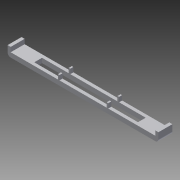
# Autodesk Inventor part: base_corner
Saved by Autodesk Inventor 2014 SP1 (Build 180222100, 222)
## iProperties
Created: 2016-08-31
Part Number: base_corner
Material: ABS Plastic
Document SubType Name: Modeling
Designer: tguillod
Density: 1.06 g/cm^3
Appearance: Smooth - White
Author: tguillod
Autodesk Inventor part; units mm, degrees
ref_plane "YZ Plane" through (0, 0, 0) normal (1, 0, 0) x (0, 1, 0)
ref_plane "XZ Plane" through (0, 0, 0) normal (0, 1, 0) x (-1, 0, 0)
ref_plane "XY Plane" through (0, 0, 0) normal (0, 0, 1) x (1, 0, 0)
sketch "Sketch1" plane through (0, 0, 0) normal (0, 0, 1) x (1, 0, 0)
  line L0 (0, 0) -> (97.5, 0)
  line L1 (97.5, 0) -> (97.5, 9)
  line L2 (97.5, 9) -> (0, 9)
  line L3 (0, 9) -> (0, 0)
  dimension "d2" = 97.5
  dimension "d3" = 9
  constraints: 8 end point, 2 parallel, 1 horizontal, 1 perpendicular
  measures "d2" distance of L1.end L2.end
  measures "d3" distance of L0.end L1.end
extrude "Extrusion1" add sketch "Sketch1" along normal blind 6
sketch "Sketch2" plane through (0, 0, 6) normal (0, 0, 1) x (1, 0, 0)
  line L0 (0, 0) -> (97.5, 0) projected
  line L1 (97.5, 0) -> (97.5, 9) projected
  line L2 (0, 9) -> (0, 0) projected
  line L3 (2, 0) -> (32.5, 0)
  line L4 (32.5, 0) -> (32.5, 9)
  line L5 (32.5, 9) -> (2, 9)
  line L6 (2, 9) -> (2, 0)
  line L7 (33.5, 9) -> (64, 9)
  line L8 (64, 9) -> (64, 0)
  line L9 (64, 0) -> (33.5, 0)
  line L10 (33.5, 0) -> (33.5, 9)
  line L11 (65, 0) -> (95.5, 0)
  line L12 (95.5, 0) -> (95.5, 9)
  line L13 (95.5, 9) -> (65, 9)
  line L14 (65, 9) -> (65, 0)
  line L15 (97.5, 9) -> (0, 9) projected
  dimension "d5" = 30.5
  dimension "d6" = 2
  dimension "d7" = 2
  dimension "d8" = 30.5
  dimension "d9" = 30.5
  dimension "d10" = 1
  constraints: 24 end point, 6 parallel, 3 collinear, 3 horizontal, 3 perpendicular, 3 point on line
  measures "d5" distance of L4.end L5.end
  measures "d6" distance between parallel lines of L6 L2
  measures "d7" distance between parallel lines of L1 L12
  measures "d8" distance of L12.end L13.end
  measures "d9" distance of L7.start L7.end
  measures "d10" distance between parallel lines of L10 L4
extrude "Extrusion2" cut sketch "Sketch2" against normal blind 3 contours L6 L5 L4 L0 | L10 L7 L8 L0 | L14 L13 L12 L0
sketch "Sketch7" plane through (0, 0, 0) normal (0, 0, -1) x (-1, 0, 0)
  line L0 (0, 0) -> (-97.5, 0) projected
  line L1 (0, 9) -> (0, 0) projected
  line L2 (-97.5, 9) -> (0, 9) projected
  line L3 (-97.5, 0) -> (-97.5, 9) projected
  line L4 (-82.25, 7) -> (-15.25, 7)
  line L5 (-15.25, 7) -> (-15.25, 2)
  line L6 (-15.25, 2) -> (-82.25, 2)
  line L7 (-82.25, 2) -> (-82.25, 7)
  line L8 (-82.25, 7) -> (-15.25, 2) construction
  line L9 (-15.25, 7) -> (-82.25, 2) construction
  line L10 (-48.75, 9) -> (-48.75, 0) construction
  line L11 (-97.5, 4.5) -> (0, 4.5) construction
  point P0 (-48.75, 4.5)
  point P1 (-48.75, 4.5)
  point P2 (-48.75, 4.5)
  dimension "d31" = 67
  dimension "d32" = 5
  constraints: 16 end point, 10 midpoint, 2 parallel, 1 horizontal, 1 perpendicular
  measures "d31" distance of L4.start L4.end
  measures "d32" distance of L4.end L5.end
extrude "Extrusion7" cut sketch "Sketch7" against normal blind 10 contours L4 L5 L6 L7
fillet "Fillet1" radius 2 2 edges at (97.5, 4.5, 0) (0, 4.5, 0)
body "Solid1"
